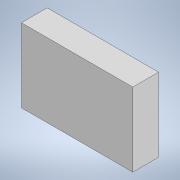
# Autodesk Inventor part: AD9833Teyleten
Saved by Autodesk Inventor 2022 (Build 260153000, 153)
## iProperties
Created: 2021-09-30
Part Number: AD9833Teyleten
Material: Generic
Document SubType Name: Modeling
Designer: iss
Density: 1 g/cm^3
Appearance: Default
Author: iss
Autodesk Inventor part; units mm, degrees
ref_plane "YZ Plane" through (0, 0, 0) normal (1, 0, 0) x (0, 1, 0)
ref_plane "XZ Plane" through (0, 0, 0) normal (0, 1, 0) x (-1, 0, 0)
ref_plane "XY Plane" through (0, 0, 0) normal (0, 0, 1) x (1, 0, 0)
sketch "Sketch1" plane through (0, 0, 0) normal (0, 0, 1) x (1, 0, 0)
  line L0 (0, 0) -> (17.272, 0)
  line L1 (17.272, 0) -> (17.272, 11.43)
  line L2 (17.272, 11.43) -> (0, 11.43)
  line L3 (0, 11.43) -> (0, 0)
  dimension "d0" = 17.272
  dimension "d1" = 11.43
  constraints: 8 end point, 2 parallel, 1 horizontal, 1 perpendicular
  measures "d0" distance of L2.end L1.end
  measures "d1" distance of L1.end L0.end
extrude "Extrusion1" add sketch "Sketch1" along normal blind 4
body "Solid1"
